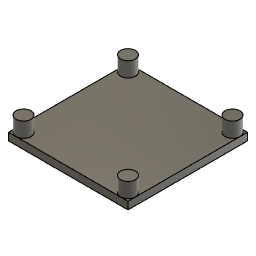
Load Plate v4 (Autodesk Fusion 360 design; units mm, degrees)
Autodesk Fusion 360 part; units mm, degrees
sketch "Sketch1" plane through (0, 0, 0) normal (0, 1, 0) x (1, 0, 0)
  line L0 (-40, -40) -> (40, -40)
  line L1 (40, -40) -> (40, 40)
  line L2 (40, 40) -> (-40, 40)
  line L3 (-40, 40) -> (-40, -40)
  constraint horizontal L0
  constraint vertical L1
  constraint horizontal L2
  constraint vertical L3
extrude "Extrude1" add sketch "Sketch1" along normal blind 5
sketch "Sketch3" plane through (0, 5, 0) normal (0, 1, 0) x (-1, 0, 0)
  line L0 (40, -40) -> (40, 40)
  line L1 (40, 40) -> (-40, 40)
  line L2 (-40, 40) -> (-40, -40)
  line L3 (-40, -40) -> (40, -40)
  circle A0 centre (35, 35) radius 5
  circle A1 centre (-35, 35) radius 5
  circle A2 centre (-35, -35) radius 5
  circle A3 centre (35, -35) radius 5
  dimension "d8" = 10
  dimension "d9" = 10
  dimension "d10" = 10
  dimension "d11" = 10
  measures "d8" diameter of A0
  measures "d9" diameter of A1
  measures "d10" diameter of A2
  measures "d11" diameter of A3
extrude "Extrude3" add sketch "Sketch3" along normal blind 10 contours A3 | A0 | A2 | A1
